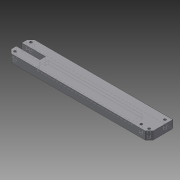
# Autodesk Inventor part: Connection Bar
Saved by Autodesk Inventor 2015 (Build 190159000, 159)
## iProperties
Created: 2019-01-11
Part Number: Connection Bar
Material: Generic
Document SubType Name: Modeling
Designer: Toby
Density: 1 g/cm^3
Appearance: Default
Author: Toby
Autodesk Inventor part; units mm, degrees
ref_plane "YZ Plane" through (0, 0, 0) normal (1, 0, 0) x (0, 1, 0)
ref_plane "XZ Plane" through (0, 0, 0) normal (0, 1, 0) x (-1, 0, 0)
ref_plane "XY Plane" through (0, 0, 0) normal (0, 0, 1) x (1, 0, 0)
sketch "Sketch1" plane through (0, 0, 0) normal (0, 0, 1) x (1, 0, 0)
  line L0 (-109.7802, 23.5714) -> (70.2198, 23.5714)
  line L1 (70.2198, 23.5714) -> (70.2198, -6.4286)
  line L2 (70.2198, -6.4286) -> (-109.7802, -6.4286)
  line L3 (-109.7802, -6.4286) -> (-109.7802, 23.5714)
  point P0 (0, 0)
  dimension "d0" = 180
  dimension "d1" = 30
  constraints: 8 end point, 2 parallel, 1 horizontal, 1 perpendicular
  measures "d0" distance of L0.start L0.end
  measures "d1" distance of L2.end L0.start
extrude "Extrusion1" add sketch "Sketch1" along normal blind 10
sketch "Sketch2" plane through (0, 0, 10) normal (0, 0, 1) x (1, 0, 0)
  line L0 (-109.7802, 23.5714) -> (-109.7802, -6.4286) projected
  line L1 (-109.7802, -6.4286) -> (70.2198, -6.4286) projected
  line L2 (70.2198, 23.5714) -> (-109.7802, 23.5714) projected
  point P0 (0, 0)
  point P1 (-104.7802, 18.5714)
  point P2 (-104.7802, -1.4286)
  dimension "d4" = 5
  dimension "d5" = 5
  dimension "d6" = 5
  dimension "d7" = 5
  measures "d4" distance from line of L0 point (-104.78, 18.571)
  measures "d5" distance from line of L0 point (-104.78, -1.429)
  measures "d6" distance from line of L1 point (-104.78, -1.429)
  measures "d7" distance from line of L2 point (-104.78, 18.571)
hole "Hole1" at (-104.7802, 18.5714, 10) at (-104.7802, -1.4286, 10) direction (0, 0, -1) diameter 3 depth 10 tip angle 118
chamfer "Chamfer1" distance 5 angle 45 2 edges at (-109.7802, 23.5714, 5) (-109.7802, -6.4286, 5)
sketch "Sketch3" plane through (0, 0, 0) normal (0, 0, -1) x (-1, 0, 0)
  line L0 (109.7802, 18.5714) -> (109.7802, -1.4286) projected
  line L1 (109.7802, 12.0714) -> (79.7802, 12.0714)
  line L2 (79.7802, 12.0714) -> (79.7802, 5.0714)
  line L3 (79.7802, 5.0714) -> (109.7802, 5.0714)
  line L4 (109.7802, 5.0714) -> (109.7802, 12.0714)
  circle A0 centre (104.7802, 18.5714) radius 1.5 projected
  circle A1 centre (104.7802, -1.4286) radius 1.5 projected
  point P0 (0, 0)
  dimension "d18" = 5
  dimension "d19" = 5
  dimension "d20" = 30
  constraints: 8 end point, 2 parallel, 1 horizontal, 1 perpendicular, 1 point on line
  measures "d18" distance edge to line of A0 L1
  measures "d19" distance edge to line of A1 L3
  measures "d20" distance between parallel lines of L0 L2
extrude "Extrusion2" cut sketch "Sketch3" against normal blind 10 contours L0 L3 L2 L1
sketch "Sketch4" plane through (0, 0, 0) normal (0, 0, -1) x (-1, 0, 0)
  line L0 (-40.2198, 15.5714) -> (79.7802, 15.5714)
  line L1 (79.7802, 15.5714) -> (79.7802, 1.5714)
  line L2 (79.7802, 1.5714) -> (-40.2198, 1.5714)
  line L3 (-40.2198, 1.5714) -> (-40.2198, 15.5714)
  line L4 (-70.2198, 23.5714) -> (104.7802, 23.5714) projected
  line L5 (-70.2198, -6.4286) -> (104.7802, -6.4286) projected
  line L6 (79.7802, 5.0714) -> (79.7802, 12.0714) projected
  line L7 (-70.2198, 23.5714) -> (-70.2198, -6.4286) projected
  point P0 (0, 0)
  dimension "d23" = 8
  dimension "d24" = 8
  dimension "d25" = 30
  constraints: 8 end point, 2 parallel, 1 collinear, 1 horizontal, 1 perpendicular
  measures "d23" distance between parallel lines of L4 L0
  measures "d24" distance between parallel lines of L5 L2
  measures "d25" distance between parallel lines of L7 L3
extrude "Extrusion3" cut sketch "Sketch4" against normal blind 4
sketch "Sketch5" plane through (0, 0, 0) normal (0, 0, -1) x (-1, 0, 0)
  line L0 (104.7802, 23.5714) -> (-70.2198, 23.5714) projected
  line L1 (-70.2198, -6.4286) -> (104.7802, -6.4286) projected
  line L2 (-70.2198, 23.5714) -> (-70.2198, -6.4286) projected
  point P0 (0, 0)
  point P1 (-65.2198, 18.5714)
  point P2 (-65.2198, -1.4286)
  point P3 (-55.2198, -1.4286)
  dimension "d28" = 5
  dimension "d29" = 5
  dimension "d30" = 5
  dimension "d31" = 5
  dimension "d32" = 5
  dimension "d33" = 10
  measures "d28" distance from line of L0 point (-65.22, 18.571)
  measures "d29" distance from line of L1 point (-65.22, -1.429)
  measures "d30" distance from line of L2 point (-65.22, -1.429)
  measures "d31" distance from line of L2 point (-65.22, 18.571)
  measures "d32" distance from line of L1 point (-55.22, -1.429)
  measures "d33" distance of point (-55.22, -1.429) point (-65.22, -1.429)
hole "Hole2" at (65.2198, 18.5714, 0) at (65.2198, -1.4286, 0) at (55.2198, -1.4286, 0) direction (0, 0, 1) diameter 3 depth 10 tip angle 118
chamfer "Chamfer2" distance 5 angle 45 1 edges at (70.2198, -6.4286, 5)
body "Solid1"
